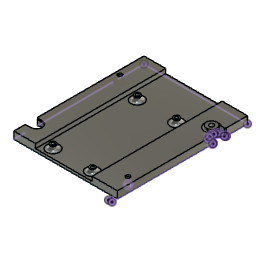
HP4957A PSU Mod v4 (Autodesk Fusion 360 design; units mm, degrees)
Autodesk Fusion 360 part; units mm, degrees
sketch "Sketch1" plane through (0, 0, 0) normal (0, 0, 1) x (1, 0, 0)
  circle A0 centre (5, 121) radius 2.5
  arc A1 (57, 153) -> (56, 153) centre (56.5, 153) ccw
  line L0 (1, 32) -> (6, 32) construction
  arc A2 (6, 19) -> (6, 32) centre (6, 25.5) ccw
  line L1 (6, 32) -> (0, 32)
  line L2 (6, 19) -> (1, 19)
  arc A3 (0, 33) -> (1, 32) centre (1, 33) ccw
  arc A4 (1, 19) -> (0, 18) centre (1, 18) ccw
  line L3 (117, 129) -> (117, 153)
  line L4 (108, 124) -> (108, 124)
  line L5 (108, 119) -> (108, 119)
  line L6 (110, 128) -> (116, 128)
  line L7 (117, 129) -> (117, 129)
  line L8 (116, 115) -> (112, 115)
  line L9 (117, 114) -> (117, 0)
  line L10 (109, 127) -> (109, 125)
  line L11 (109, 118) -> (109, 116)
  arc A5 (108, 124) -> (108, 119) centre (108, 121.5) ccw
  line L12 (112, 115) -> (110, 115)
  arc A6 (108, 124) -> (109, 125) centre (108, 125) ccw
  arc A7 (109, 118) -> (108, 119) centre (108, 118) ccw
  arc A8 (110, 128) -> (109, 127) centre (110, 127) ccw
  arc A9 (109, 116) -> (110, 115) centre (110, 116) ccw
  arc A10 (117, 114) -> (116, 115) centre (116, 114) ccw
  arc A11 (116, 128) -> (117, 129) centre (116, 129) ccw
  circle A12 centre (109, 26) radius 2.5
  line L13 (117, 0) -> (0, 0)
  line L14 (0, 0) -> (0, 18)
  line L15 (0, 153) -> (117, 153)
  line L16 (0, 33) -> (0, 153)
  dimension "d2" = 153
  dimension "d5" = 5
  dimension "d18" = 1
  dimension "d19" = 1
  dimension "d82" = 5
  dimension "d83" = 1
  dimension "d84" = 1
  dimension "d85" = 1
  dimension "d87" = 5
  constraint coincident L1.end L0
  constraint tangent L0 A3
  constraint tangent L2 A4
  constraint perpendicular L6 L10
  constraint perpendicular L8 L9
  constraint collinear L10 L11
  constraint perpendicular L9 L12
  constraint tangent L10 A6
  constraint tangent L11 A7
  constraint tangent L6 A8
  constraint tangent L10 A8
  constraint tangent L11 A9
  constraint tangent L12 A9
  constraint equal A8 A9
  constraint tangent L8 A10
  constraint tangent L9 A10
  constraint equal A8 A10
  constraint tangent L6 A11
  constraint equal A8 A11
  constraint coincident L13.end L14.start
  constraint perpendicular L9 L13
  constraint tangent A4 L14
  constraint perpendicular L3 L15
  constraint tangent A3 L16
  measures "d2" distance of L13.end L15.start
  measures "d5" diameter of A0
  measures "d18" radius of A3
  measures "d19" radius of A4
  measures "d82" diameter of A5
  measures "d83" radius of A6
  measures "d84" radius of A7
  measures "d85" radius of A8
  measures "d87" diameter of A12
extrude "Extrude1" add sketch "Sketch1" against normal blind 8 contours A2 L1 L2 A3 A4 L3 L6 L8 L9 L10 L11 A5 L12 A6 A7 A8 A9 A10 A11 L13 L14 L15 L16
cylinder "CylinderPrimitive5" cut diameter 12 height -6.4 placed x (0, 1, 0) y (1, 0, 0) z (0, 0, -1) at (5, 121, -8)
cylinder "CylinderPrimitive6" cut diameter 18 height -6.4 placed x (0, 1, 0) y (1, 0, 0) z (0, 0, -1) at (6, 25.5, -8)
box "BoxPrimitive1" cut length 6 width 113 height -8 placed x (0, 1, 0) y (-1, 0, 0) z (0, 0, 1) at (113, 0, 0)
sketch "Sketch9" plane through (0, 0, 0) normal (0, 0, 1) x (-1, 0, 0)
  line L0 (0, -6) -> (-113, -6)
  arc A0 (0, -33) -> (-1, -32) centre (-1, -33) ccw
  line L1 (-1, -32) -> (-6, -32)
  arc A1 (-6, -19) -> (-6, -32) centre (-6, -25.5) ccw
  line L2 (-6, -19) -> (-1, -19)
  arc A2 (-1, -19) -> (0, -18) centre (-1, -18) ccw
  circle A3 centre (-5, -121) radius 2.5
  line L3 (-88.5, -6) -> (-88.5, -153) construction
  line L4 (-24.5, -6) -> (-24.5, -153) construction
  line L5 (-24.5, -6) -> (-88.5, -6)
  line L6 (-88.5, -6) -> (-88.5, -153)
  line L7 (-88.5, -153) -> (-24.5, -153)
  line L8 (-24.5, -153) -> (-24.5, -6)
  circle A4 centre (-34.275, -111.25) radius 1.75
  circle A5 centre (-34.275, -16) radius 1.75
  circle A6 centre (-78.725, -16) radius 1.75
  circle A7 centre (-78.725, -111.25) radius 1.75
  circle A8 centre (-34.275, -16) radius 3.25
  circle A9 centre (-34.275, -111.25) radius 3.25
  circle A10 centre (-78.725, -111.25) radius 3.25
  circle A11 centre (-78.725, -16) radius 3.25
  line L9 (-113, -6) -> (-113, 0)
  line L10 (-113, 0) -> (-117, 0)
  line L11 (-117, 0) -> (-117, -114)
  arc A12 (-117, -114) -> (-116, -115) centre (-116, -114) ccw
  line L12 (-116, -115) -> (-110, -115)
  arc A13 (-109, -116) -> (-110, -115) centre (-110, -116) ccw
  arc A14 (-110, -128) -> (-109, -127) centre (-110, -127) ccw
  line L13 (-110, -128) -> (-116, -128)
  arc A15 (-116, -128) -> (-117, -129) centre (-116, -129) ccw
  line L14 (-117, -129) -> (-117, -153)
  line L15 (-117, -153) -> (0, -153)
  line L16 (0, -153) -> (0, -33)
  line L17 (0, -18) -> (0, -6)
  line L18 (-109, -116) -> (-109, -118)
  arc A16 (-109, -118) -> (-108, -119) centre (-108, -118) ccw
  arc A17 (-108, -124) -> (-108, -119) centre (-108, -121.5) ccw
  arc A18 (-108, -124) -> (-109, -125) centre (-108, -125) ccw
  line L19 (-109, -125) -> (-109, -127)
  circle A19 centre (-109, -26) radius 2.5
  dimension "d53" = 3.5
  dimension "d54" = 3.5
  dimension "d55" = 3.5
  dimension "d56" = 3.5
  dimension "d57" = 6.5
  dimension "d58" = 6.5
  dimension "d59" = 6.5
  dimension "d60" = 6.5
  constraint horizontal L5
  constraint vertical L6
  constraint horizontal L7
  constraint vertical L8
  constraint concentric A5 A8
  constraint concentric A4 A9
  constraint concentric A7 A10
  constraint concentric A6 A11
  measures "d53" diameter of A4
  measures "d54" diameter of A5
  measures "d55" diameter of A6
  measures "d56" diameter of A7
  measures "d57" diameter of A8
  measures "d58" diameter of A9
  measures "d59" diameter of A10
  measures "d60" diameter of A11
extrude "Extrude2" cut sketch "Sketch9" against normal blind 5 contours L0 L5 L6 L7 L8 L15 | A4 | A5 | A6 | A7
move_face "OffsetFaces1" offset -1 1 faces at (75.9871, 16.1615, 0)
fillet "Fillet2" radius 4 4 edges at (37.3051, 17.1753, -5) (37.3051, 112.4253, -5) (81.7551, 112.4253, -5) (81.7551, 17.1753, -5)
cylinder "CylinderPrimitive7" cut diameter 3 height -110 placed x (1, 0, 0) y (0, 1, 0) z (0, 0, 1) at (34.275, 16, 0)
cylinder "CylinderPrimitive8" cut diameter 3 height -10 placed x (1, 0, 0) y (0, 1, 0) z (0, 0, 1) at (34.275, 111.25, 0)
cylinder "CylinderPrimitive9" cut diameter 3 height -10 placed x (1, 0, 0) y (0, 1, 0) z (0, 0, 1) at (78.725, 16, -1)
cylinder "CylinderPrimitive10" cut diameter 3 height -10 placed x (1, 0, 0) y (0, 1, 0) z (0, 0, 1) at (78.725, 111.25, 0)
sketch "Sketch14" plane through (0, 0, -8) normal (0, 0, -1) x (1, 0, 0)
  circle A0 centre (78.725, -111.25) radius 1.5
  circle A1 centre (78.725, -16) radius 1.5
  circle A2 centre (34.275, -111.25) radius 1.5
  circle A3 centre (34.275, -16) radius 1.5
  line L0 (113, -6) -> (0, -6)
  arc A4 (0, -18) -> (0.2084, -18.6111) centre (1, -18) ccw
  arc A5 (0.2084, -32.3889) -> (0.2084, -18.6111) centre (6, -25.5) ccw
  arc A6 (0.2084, -32.3889) -> (0, -33) centre (1, -33) ccw
  arc A7 (0, -124.3166) -> (0, -117.6834) centre (5, -121) ccw
  line L1 (113, 0) -> (113, -6)
  line L2 (0, -6) -> (0, -18)
  line L3 (0, -33) -> (0, -117.6834)
  line L4 (0, -124.3166) -> (0, -153)
  line L5 (0, -153) -> (117, -153)
  line L6 (117, -153) -> (117, -129)
  arc A8 (117, -129) -> (116, -128) centre (116, -129) ccw
  line L7 (116, -128) -> (110, -128)
  arc A9 (109, -127) -> (110, -128) centre (110, -127) ccw
  line L8 (109, -127) -> (109, -125)
  line L9 (109, -118) -> (109, -116)
  arc A10 (110, -115) -> (109, -116) centre (110, -116) ccw
  line L10 (110, -115) -> (116, -115)
  arc A11 (116, -115) -> (117, -114) centre (116, -114) ccw
  line L11 (117, -114) -> (117, 0)
  line L12 (117, 0) -> (113, 0)
  arc A12 (109, -125) -> (108, -124) centre (108, -125) ccw
  arc A13 (108, -119) -> (108, -124) centre (108, -121.5) ccw
  arc A14 (108, -119) -> (109, -118) centre (108, -118) ccw
  circle A15 centre (109, -26) radius 2.5
sketch "Sketch15" plane through (0, 0, -8) normal (0, 0, -1) x (1, 0, 0)
  circle A0 centre (78.725, -16) radius 1.75
  circle A1 centre (34.275, -16) radius 1.75
  circle A2 centre (78.725, -111.25) radius 1.75
  circle A3 centre (34.275, -111.25) radius 1.75
  line L0 (35.9204, -18.85) -> (37.5659, -16)
  line L1 (37.5659, -16) -> (35.9204, -13.15)
  line L2 (35.9204, -13.15) -> (32.6296, -13.15)
  line L3 (32.6296, -13.15) -> (30.9841, -16)
  line L4 (30.9841, -16) -> (32.6296, -18.85)
  line L5 (32.6296, -18.85) -> (35.9204, -18.85)
  line L6 (32.6296, -108.4) -> (30.9841, -111.25)
  line L7 (30.9841, -111.25) -> (32.6296, -114.1)
  line L8 (32.6296, -114.1) -> (35.9204, -114.1)
  line L9 (35.9204, -114.1) -> (37.5659, -111.25)
  line L10 (37.5659, -111.25) -> (35.9204, -108.4)
  line L11 (35.9204, -108.4) -> (32.6296, -108.4)
  line L12 (80.3704, -18.85) -> (82.0159, -16)
  line L13 (82.0159, -16) -> (80.3704, -13.15)
  line L14 (80.3704, -13.15) -> (77.0796, -13.15)
  line L15 (77.0796, -13.15) -> (75.4341, -16)
  line L16 (75.4341, -16) -> (77.0796, -18.85)
  line L17 (77.0796, -18.85) -> (80.3704, -18.85)
  line L18 (77.0796, -108.4) -> (75.4341, -111.25)
  line L19 (75.4341, -111.25) -> (77.0796, -114.1)
  line L20 (77.0796, -114.1) -> (80.3704, -114.1)
  line L21 (80.3704, -114.1) -> (82.0159, -111.25)
  line L22 (82.0159, -111.25) -> (80.3704, -108.4)
  line L23 (80.3704, -108.4) -> (77.0796, -108.4)
  point P0 (78.725, -16)
  point P1 (78.725, -111.25)
  point P2 (34.275, -16)
  point P3 (34.275, -111.25)
  point P4 (34.275, -16)
  point P5 (34.275, -111.25)
  point P6 (78.725, -16)
  point P7 (78.725, -111.25)
  dimension "d103" = 2.85
  dimension "d104" = 2.85
  dimension "d105" = 2.85
  dimension "d106" = 2.85
  constraint coincident P6 P0
  constraint coincident P7 P1
  constraint coincident P4 A1.centre
  constraint coincident P5 P3
  measures "d103" distance of P4 L5
  measures "d104" distance of P5 L11
  measures "d105" distance of P6 L17
  measures "d106" distance of P7 L23
extrude "Extrude3" cut sketch "Sketch15" against normal blind 3 contours A0 | A1 | A2 | A3 | L0 L1 L2 L3 L4 L5 | L6 L7 L8 L9 L10 L11 | L12 L13 L14 L15 L16 L17 | L18 L19 L20 L21 L22 L23
box "BoxPrimitive2" cut length 16 width 11 height -9 placed x (0, 1, 0) y (-1, 0, 0) z (0, 0, 1) at (124, -10, 0)
cylinder "CylinderPrimitive11" cut diameter 12 height -6.4 placed x (0, 1, 0) y (1, 0, 0) z (0, 0, -1) at (109, 26, -8)
cylinder "CylinderPrimitive12" cut diameter 12 height -6.4 placed x (0, 1, 0) y (1, 0, 0) z (0, 0, -1) at (108, 121.5, -8)
cylinder "CylinderPrimitive13" add diameter 12 height 2 placed x (1, 0, 0) y (0, 1, 0) z (0, 0, 1) at (108, 121.5, 0)
cylinder "CylinderPrimitive14" cut diameter 5 height -2 placed x (1, 0, 0) y (0, 1, 0) z (0, 0, 1) at (108, 121.5, 2)
fillet "Fillet3" radius 2 1 edges at (102, 121.5, 0)
